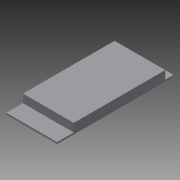
# Autodesk Inventor part: button
Saved by Autodesk Inventor 2015 (Build 190159000, 159)
## iProperties
Created: 2020-03-18
Part Number: button
Material: Generic
Document SubType Name: Modeling
Designer: Toby
Density: 1 g/cm^3
Appearance: Default
Author: Toby
Autodesk Inventor part; units mm, degrees
ref_plane "YZ Plane" through (0, 0, 0) normal (1, 0, 0) x (0, 1, 0)
ref_plane "XZ Plane" through (0, 0, 0) normal (0, 1, 0) x (-1, 0, 0)
ref_plane "XY Plane" through (0, 0, 0) normal (0, 0, 1) x (1, 0, 0)
sketch "Sketch1" plane through (0, 0, 0) normal (0, 0, 1) x (1, 0, 0)
  line L0 (-9.4085, 11.4915) -> (2.7915, 11.4915)
  line L1 (2.7915, 11.4915) -> (2.7915, -10.5085)
  line L2 (2.7915, -10.5085) -> (-9.4085, -10.5085)
  line L3 (-9.4085, -10.5085) -> (-9.4085, 11.4915)
  point P0 (0, 0)
  dimension "d0" = 22
  dimension "d1" = 12.2
  constraints: 8 end point, 2 parallel, 1 horizontal, 1 perpendicular
  measures "d0" distance of L2.end L0.start
  measures "d1" distance of L0.start L0.end
extrude "Extrusion1" add sketch "Sketch1" along normal blind 2
sketch "Sketch2" plane through (0, 0, 0) normal (0, 0, -1) x (-1, 0, 0)
  line L0 (-2.7915, -14.5085) -> (9.4085, -14.5085)
  line L1 (9.4085, -14.5085) -> (9.4085, 13.4915)
  line L2 (9.4085, 13.4915) -> (-2.7915, 13.4915)
  line L3 (-2.7915, 13.4915) -> (-2.7915, -14.5085)
  line L4 (9.4085, -10.5085) -> (9.4085, 11.4915) projected
  line L5 (-2.7915, 11.4915) -> (-2.7915, -10.5085) projected
  line L6 (9.4085, 11.4915) -> (-2.7915, 11.4915) projected
  line L7 (-2.7915, -10.5085) -> (9.4085, -10.5085) projected
  point P0 (0, 0)
  dimension "d4" = 2
  dimension "d5" = 4
  constraints: 8 end point, 2 collinear, 2 parallel, 1 horizontal, 1 perpendicular
  measures "d4" distance between parallel lines of L6 L2
  measures "d5" distance between parallel lines of L0 L7
extrude "Extrusion2" add sketch "Sketch2" along normal blind 0.4
body "Solid1"
